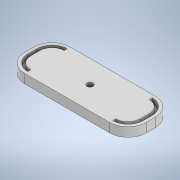
# Autodesk Inventor part: base
Saved by Autodesk Inventor 2022 (Build 260153000, 153)
## iProperties
Created: 2022-04-05
Part Number: base
Material: Genérico
Document SubType Name: Modeling
Designer: User
Density: 1 g/cm^3
Appearance: Valor por defecto
Author: User
Autodesk Inventor part; units mm, degrees
ref_plane "YZ Plane" through (0, 0, 0) normal (1, 0, 0) x (0, 1, 0)
ref_plane "XZ Plane" through (0, 0, 0) normal (0, 1, 0) x (-1, 0, 0)
ref_plane "XY Plane" through (0, 0, 0) normal (0, 0, 1) x (1, 0, 0)
sketch "Boceto1" plane through (0, 0, 0) normal (0, 1, 0) x (-1, 0, 0)
  line L0 (140, 75) -> (-140, 75)
  line L1 (-200, 15) -> (-200, -15)
  line L2 (-140, -75) -> (140, -75)
  arc A0 (-140, 75) -> (-200, 15) centre (-140, 15) ccw
  arc A1 (-200, -15) -> (-140, -75) centre (-140, -15) ccw
  line L3 (-140, 65) -> (-140, 55)
  line L4 (-140, -55) -> (-140, -65)
  arc A2 (-140, 65) -> (-190, 15) centre (-140, 15) ccw
  line L5 (-190, 15) -> (-190, -15)
  arc A3 (-190, -15) -> (-140, -65) centre (-140, -15) ccw
  arc A4 (-140, 55) -> (-180, 15) centre (-140, 15) ccw
  line L6 (-180, 15) -> (-180, -15)
  arc A5 (-180, -15) -> (-140, -55) centre (-140, -15) ccw
  line L7 (140, 65) -> (140, 55)
  line L8 (140, -55) -> (140, -65)
  arc A6 (190, 15) -> (140, 65) centre (140, 15) ccw
  line L9 (190, 15) -> (190, -15)
  arc A7 (140, -65) -> (190, -15) centre (140, -15) ccw
  arc A8 (180, 15) -> (140, 55) centre (140, 15) ccw
  line L10 (180, 15) -> (180, -15)
  arc A9 (140, -55) -> (180, -15) centre (140, -15) ccw
  line L11 (200, 15) -> (200, -15)
  arc A10 (200, 15) -> (140, 75) centre (140, 15) ccw
  arc A11 (140, -75) -> (200, -15) centre (140, -15) ccw
  circle A12 centre (0, 0) radius 10
  constraints: 24 end point, 24 point on circle, 13 centre point, 4 tangent, 2 vertical, 1 coincident, 1 horizontal, 1 parallel, 1 perpendicular, 4 other
extrude "Extrusión1" add sketch "Boceto1" along normal blind 15 contours A6 L9 A7 L8 A9 L10 A8 L7
extrude "Extrusión2" add sketch "Boceto1" along normal blind 15 contours L3 A4 L6 A5 L4 A3 L5 A2
extrude "Extrusión3" add sketch "Boceto1" along normal blind 30
extrude "Extrusión4" add sketch "Boceto1" along normal blind 10 contours A12
hole "Agujero1" at (0, 0, 0) direction (0, 1, 0) diameter 3 end through all
